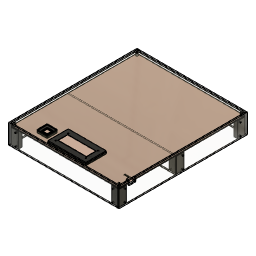
Case (Autodesk Fusion 360 design; units mm, degrees)
Autodesk Fusion 360 part; units mm, degrees
(part 1 of 2)
sketch "Sketch1" plane through (0, 0, 0) normal (0, 0, 1) x (1, 0, 0) in component "PCB"
  line L0 (-131, 153.5) -> (131, 153.5) construction
  line L1 (131, 153.5) -> (131, -153.5) construction
  line L2 (131, -153.5) -> (-131, -153.5) construction
  line L3 (-131, -153.5) -> (-131, 153.5) construction
  line L4 (-131, 153.5) -> (131, -153.5) construction
  line L5 (131, 153.5) -> (-131, -153.5) construction
  line L6 (-135, 157.5) -> (135, 157.5)
  line L7 (135, 157.5) -> (135, -157.5)
  line L8 (135, -157.5) -> (-135, -157.5)
  line L9 (-135, -157.5) -> (-135, 157.5)
  line L10 (-135, 157.5) -> (135, -157.5) construction
  line L11 (135, 157.5) -> (-135, -157.5) construction
  circle A0 centre (-131, 153.5) radius 1.6
  circle A1 centre (131, 153.5) radius 1.6
  circle A2 centre (-131, -153.5) radius 1.6
  circle A3 centre (131, -153.5) radius 1.6
  line L12 (135, -127.52) -> (128, -127.52) construction
  line L13 (128, -127.52) -> (128, -123.02)
  line L14 (128, -123.02) -> (135, -123.02)
  line L15 (128, -132.02) -> (135, -132.02)
  line L16 (128, -127.52) -> (128, -132.02)
  line L17 (122.64, -122.688) -> (112.36, -122.688)
  line L18 (112.36, -122.688) -> (112.36, -120.028)
  line L19 (112.36, -120.028) -> (122.64, -120.028)
  line L20 (122.64, -120.028) -> (122.64, -122.688)
  line L21 (122.64, -122.688) -> (112.36, -120.028) construction
  line L22 (112.36, -122.688) -> (122.64, -120.028) construction
  circle A4 centre (113.69, -121.358) radius 0.5
  circle A5 centre (116.23, -121.358) radius 0.5
  circle A6 centre (118.77, -121.358) radius 0.5
  circle A7 centre (121.31, -121.358) radius 0.5
  line L23 (113.69, -121.358) -> (116.23, -121.358) construction
  line L24 (116.23, -121.358) -> (118.77, -121.358) construction
  line L25 (118.77, -121.358) -> (121.31, -121.358) construction
  line L26 (121.31, -121.358) -> (122.64, -121.358) construction
  line L27 (113.69, -121.358) -> (112.36, -121.358) construction
  line L28 (-40, -109.858) -> (40, -109.858)
  line L29 (40, -109.858) -> (40, -145.858)
  line L30 (40, -145.858) -> (-40, -145.858)
  line L31 (-40, -145.858) -> (-40, -109.858)
  line L32 (-40, -109.858) -> (40, -145.858) construction
  line L33 (40, -109.858) -> (-40, -145.858) construction
  line L34 (-35.35, -115.958) -> (35.35, -115.958)
  line L35 (35.35, -115.958) -> (35.35, -139.758)
  line L36 (35.35, -139.758) -> (-35.35, -139.758)
  line L37 (-35.35, -139.758) -> (-35.35, -115.958)
  line L38 (-35.35, -115.958) -> (35.35, -139.758) construction
  line L39 (35.35, -115.958) -> (-35.35, -139.758) construction
  line L40 (-37.7, -112.158) -> (37.7, -112.158) construction
  line L41 (37.7, -112.158) -> (37.7, -143.558) construction
  line L42 (37.7, -143.558) -> (-37.7, -143.558) construction
  line L43 (-37.7, -143.558) -> (-37.7, -112.158) construction
  line L44 (-37.7, -112.158) -> (37.7, -143.558) construction
  line L45 (37.7, -112.158) -> (-37.7, -143.558) construction
  circle A8 centre (-37.7, -112.158) radius 1.4
  circle A9 centre (37.7, -112.158) radius 1.4
  circle A10 centre (37.7, -143.558) radius 1.4
  circle A11 centre (-37.7, -143.558) radius 1.4
  point P0 (117.5, -121.358)
  point P1 (0, -127.858)
  point P2 (0, -127.858)
  point P3 (0, -127.858)
  dimension "d1" = 262
  dimension "d2" = 307
  dimension "d3" = 270
  dimension "d4" = 315
  dimension "d5" = 3.2
  dimension "d8" = 29.98
  dimension "d9" = 9
  dimension "d10" = 7
  dimension "d17" = 10.28
  dimension "d18" = 2.66
  dimension "d19" = 2.54
  dimension "d20" = 1
  dimension "d21" = 36.142
  dimension "d22" = 17.5
  dimension "d30" = 29.642
  dimension "d31" = 135
  dimension "d32" = 80
  dimension "d33" = 36
  dimension "d34" = 70.7
  dimension "d35" = 23.8
  dimension "d279" = 75.4
  dimension "d280" = 31.4
  dimension "d281" = 2.8
  constraint horizontal L0
  constraint perpendicular L0 L1
  constraint parallel L0 L2
  constraint parallel L1 L3
  constraint coincident L4 origin
  constraint coincident L5 origin
  constraint horizontal L6
  constraint perpendicular L6 L7
  constraint parallel L6 L8
  constraint parallel L7 L9
  constraint coincident L10 origin
  constraint coincident L11 origin
  constraint coincident L0.start L3.end
  constraint coincident L0.end L1.start
  constraint coincident L2.end L3.start
  constraint coincident L1.end L2.start
  constraint equal A1 A3
  constraint equal A2 A3
  constraint equal A0 A2
  constraint coincident L7 L12.start
  constraint perpendicular L1 L12
  constraint perpendicular L12 L13
  constraint coincident L7 L14.end
  constraint perpendicular L7 L14
  constraint symmetric L13.start L12 L16.start
  constraint symmetric L12 L13.end L15.start
  constraint symmetric L12 L14.end L15.end
  constraint horizontal L17
  constraint perpendicular L17 L18
  constraint parallel L17 L19
  constraint parallel L18 L20
  constraint coincident L21 P0
  constraint coincident L22 P0
  constraint coincident A4.centre L23.start
  constraint horizontal L23
  constraint coincident A5.centre L23.end
  constraint equal A4 A5
  constraint equal A5 A6
  constraint equal A6 A7
  constraint parallel L23 L24
  constraint parallel L23 L25
  constraint parallel L25 L26
  constraint coincident A6.centre L24.end
  constraint coincident A7.centre L25.end
  constraint equal L23 L24
  constraint equal L24 L25
  constraint parallel L23 L27
  constraint equal L26 L27
  constraint midpoint L18 L27.end
  constraint midpoint L20 L26.end
  constraint horizontal L28
  constraint perpendicular L28 L29
  constraint parallel L28 L30
  constraint parallel L29 L31
  constraint coincident L32 P3
  constraint coincident L33 P3
  constraint horizontal L34
  constraint perpendicular L34 L35
  constraint parallel L34 L36
  constraint parallel L35 L37
  constraint coincident L38 P3
  constraint coincident L39 P3
  constraint coincident P3 P2
  constraint horizontal L40
  constraint perpendicular L40 L41
  constraint parallel L40 L42
  constraint parallel L41 L43
  constraint coincident L44 P3
  constraint coincident L45 P3
  constraint coincident L40.start L43.end
  constraint coincident L40.end L41.start
  constraint coincident L41.end L42.start
  constraint coincident L42.end L43.start
  constraint equal A8 A11
  constraint equal A8 A9
  constraint equal A9 A10
  measures "d1" distance of L1.end L2.end
  measures "d2" distance of L0.end L1.end
  measures "d3" distance of L7.end L8.end
  measures "d4" distance of L6.end L7.end
  measures "d5" diameter of A0
  measures "d8" distance of L7.end L12.start
  measures "d9" distance of L14 L15
  measures "d10" distance of L13.end L14.end
  measures "d17" distance of L18.end L19.end
  measures "d18" distance of L17.end L18.end
  measures "d19" distance of A4.centre A5.centre
  measures "d20" diameter of A7
  measures "d21" distance of L8 P0
  measures "d22" distance of L7 P0
  measures "d30" distance of L8 P3
  measures "d31" distance of L9 P3
  measures "d32" distance of L28.start L28.end
  measures "d33" distance of L28.end L29.end
  measures "d34" distance of L35.end L36.end
  measures "d35" distance of L34.end L35.end
  measures "d279" distance of L41.end L42.end
  measures "d280" distance of L40.end L41.end
  measures "d281" diameter of A8
extrude "Extrude1" add sketch "Sketch1" along normal blind 1.6 contours L6 L7 L8 L9 L13 L14 L15 L16 makes body 1 in component "PCB"
extrude "Extrude2" add sketch "Sketch1" along normal blind 5 contours L7 L13 L14 L15 L16 bodies 1 in component "PCB"
extrude "Extrude3" add sketch "Sketch1" along normal blind 4 contours L28 L29 L30 L31 bodies 1 in component "PCB"
extrude "Extrude4" add sketch "Sketch1" along normal blind 11 contours L34 L35 L36 L37 bodies 1 in component "PCB"
sketch "Sketch1 (2)" plane through (0, 0, 0) normal (0, 0, 1) x (1, 0, 0) in component "Corner"
  circle A0 centre (0, 0) radius 2.3
  line L0 (0, 0) -> (0, -9.2) construction
  line L1 (0, 0) -> (9.2, 0) construction
  circle A1 centre (0, -9.2) radius 2.3
  circle A2 centre (9.2, 0) radius 2.3
  line L2 (-4.6, 4.6) -> (-4.6, -13.8)
  line L3 (-4.6, -13.8) -> (4.6, -13.8)
  line L4 (4.6, -13.8) -> (4.6, -4.6)
  line L5 (4.6, -4.6) -> (13.8, -4.6)
  line L6 (13.8, -4.6) -> (13.8, 4.6)
  line L7 (13.8, 4.6) -> (-4.6, 4.6)
  line L8 (4.6, 0) -> (4.6, 4.6) construction
  line L9 (4.6, 0) -> (4.6, -4.6) construction
  line L10 (0, -4.6) -> (4.6, -4.6) construction
  line L11 (0, -4.6) -> (-4.6, -4.6) construction
  line L12 (9.2, 0) -> (13.8, 0) construction
  line L13 (0, -9.2) -> (0, -13.8) construction
  dimension "d41" = 4.6
  dimension "d42" = 9.2
  dimension "d43" = 4.6
  dimension "d44" = 4.6
  constraint coincident A0.centre L0.start
  constraint vertical L0
  constraint perpendicular L0 L1
  constraint equal L0 L1
  constraint coincident L0.end A1.centre
  constraint coincident L1.end A2.centre
  constraint equal A0 A2
  constraint equal A1 A2
  constraint vertical L2
  constraint perpendicular L2 L3
  constraint perpendicular L3 L4
  constraint perpendicular L4 L5
  constraint perpendicular L5 L6
  constraint perpendicular L6 L7
  constraint coincident L2.start L7.end
  constraint midpoint L1 L8.start
  constraint coincident L7 L8.end
  constraint perpendicular L7 L8
  constraint coincident L5 L4.end
  constraint perpendicular L5 L9
  constraint midpoint L0 L10.start
  constraint coincident L4 L5.start
  constraint perpendicular L4 L10
  constraint coincident L2 L11.end
  constraint perpendicular L2 L11
  constraint coincident L4.end L5.start
  constraint midpoint L6 L12.end
  constraint midpoint L3 L13.end
  constraint equal L11 L13
  constraint equal L12 L13
  measures "d41" diameter of A0
  measures "d42" distance of A0.centre L0.end
  measures "d43" distance of L8.start L8.end
  measures "d44" distance of L10.start L11.end
extrude "Extrude1'" add sketch "Sketch1 (2)" along normal blind 9 separate body contours A1 | A2 | L2 L3 L4 L5 L6 L7 makes body 2 in component "Corner"
extrude "Extrude2'" add sketch "Sketch1 (2)" along normal blind 3 contours A0 bodies 2 in component "Corner"
sketch "Sketch2" plane through (-4.6, 0, 0) normal (-1, 0, 0) x (0, -1, 0) in component "Corner"
  line L0 (-4.6, 0) -> (13.8, 0)
  line L1 (13.8, 0) -> (13.8, 9)
  line L2 (13.8, 9) -> (-4.6, 9)
  line L3 (-4.6, 9) -> (-4.6, 0)
  line L4 (11.5, 0) -> (6.9, 0)
  line L5 (13.8, 4.5) -> (9.2, 4.5) construction
  line L6 (9.2, 0) -> (9.2, 4.5) construction
  circle A0 centre (9.2, 4.5) radius 1.45
  dimension "d49" = 2.9
  constraint midpoint L1 L5.start
  constraint perpendicular L1 L5
  constraint midpoint L4 L6.start
  constraint perpendicular L4 L6
  constraint coincident L5.end L6.end
  measures "d49" diameter of A0
extrude "Extrude3'" cut sketch "Sketch2" against normal blind 6 contours A0 bodies 2 in component "Corner"
sketch "Sketch3" plane through (0, 4.6, 0) normal (0, 1, 0) x (-1, 0, 0) in component "Corner"
  line L0 (-13.8, 0) -> (4.6, 0)
  line L1 (4.6, 0) -> (4.6, 9)
  line L2 (4.6, 9) -> (-13.8, 9)
  line L3 (-13.8, 9) -> (-13.8, 0)
  line L4 (-6.9, 0) -> (-11.5, 0)
  line L5 (-13.8, 4.5) -> (-9.2, 4.5) construction
  line L6 (-9.2, 0) -> (-9.2, 4.5) construction
  circle A0 centre (-9.2, 4.5) radius 1.45
  dimension "d52" = 2.9
  constraint midpoint L3 L5.start
  constraint perpendicular L3 L5
  constraint midpoint L4 L6.start
  constraint perpendicular L4 L6
  constraint coincident L5.end L6.end
  measures "d52" diameter of A0
extrude "Extrude4'" cut sketch "Sketch3" against normal blind 6 contours A0 bodies 2 in component "Corner"
sketch "Sketch1 (3)" plane through (0, 0, 0) normal (0, 0, 1) x (1, 0, 0) in component "Washer"
  circle A0 centre (0, 0) radius 1.6
  circle A1 centre (0, 0) radius 2.6
  dimension "d55" = 3.2
  dimension "d56" = 1
  constraint coincident A0.centre A1.centre
  measures "d55" diameter of A0
extrude "Extrude1''" add sketch "Sketch1 (3)" along normal blind 1 separate body makes body 3 in component "Washer"
sketch "Sketch1 (4)" plane through (0, 0, 0) normal (0, 0, 1) x (1, 0, 0) in component "PlateWasher"
  circle A0 centre (0, 0) radius 1.6
  circle A1 centre (0, 0) radius 2.6
  dimension "d59" = 3.2
  dimension "d60" = 1
  constraint coincident A0.centre A1.centre
  measures "d59" diameter of A0
extrude "Extrude1'''" add sketch "Sketch1 (4)" along normal blind 4 separate body makes body 4 in component "PlateWasher"
move_face "OffsetFaces1" offset 30 1 faces at (4.6, 1.5333, 0) on bodies 2 in component "Corner"
sketch "Sketch5" plane through (0, 4.6, 0) normal (0, 1, 0) x (-1, 0, 0) in component "Corner"
  circle A0 centre (-9.2, 4.5) radius 1.45
  line L0 (-13.8, -30) -> (4.6, -30)
  line L1 (4.6, -30) -> (4.6, 9)
  line L2 (4.6, 9) -> (-13.8, 9)
  line L3 (-13.8, 9) -> (-13.8, -30)
  line L4 (-9.2, 4.5) -> (-9.2, 9) construction
  line L5 (-9.2, -30) -> (-9.2, -25.5) construction
  circle A1 centre (-9.2, -25.5) radius 1.45
  line L6 (-9.2, -25.5) -> (-9.2, 4.5) construction
  constraint coincident A0.centre L4.start
  constraint coincident L2 L4.end
  constraint perpendicular L2 L4
  constraint coincident L0 L5.start
  constraint perpendicular L0 L5
  constraint coincident L5.end A1.centre
  constraint equal A0 A1
  constraint equal L4 L5
  constraint vertical L6
extrude "Extrude6" cut sketch "Sketch5" against normal up to surface (6 mm away) contours A1 bodies 2 in component "Corner"
sketch "Sketch6" plane through (-4.6, 0, 0) normal (-1, 0, 0) x (0, -1, 0) in component "Corner"
  circle A0 centre (9.2, 4.5) radius 1.45
  line L0 (-4.6, -30) -> (13.8, -30)
  line L1 (13.8, -30) -> (13.8, 9)
  line L2 (13.8, 9) -> (-4.6, 9)
  line L3 (-4.6, 9) -> (-4.6, -30)
  line L4 (9.2, 4.5) -> (9.2, 9) construction
  line L5 (9.2, -30) -> (9.2, -25.5) construction
  line L6 (9.2, -25.5) -> (9.2, 4.5) construction
  circle A1 centre (9.2, -25.5) radius 1.45
  constraint coincident A0.centre L4.start
  constraint coincident L2 L4.end
  constraint perpendicular L2 L4
  constraint coincident L0 L5.start
  constraint perpendicular L0 L5
  constraint parallel L4 L6
  constraint equal L4 L5
  constraint coincident L5.end L6.start
  constraint equal A0 A1
extrude "Extrude7" cut sketch "Sketch6" against normal up to surface (6 mm away) contours A1 bodies 2 in component "Corner"
sketch "Sketch1 (5)" plane through (0, -158.1, 0) normal (0, -1, 0) x (1, 0, 0) in component "Panel1"
  circle A0 centre (-121.8, -35.5) radius 1.45
  circle A1 centre (-121.8, -5.5) radius 1.45
  line L0 (-135.6, -40) -> (-117.2, -40)
  line L1 (-117.2, -40) -> (-117.2, -1)
  line L2 (-117.2, -1) -> (-135.6, -1)
  line L3 (-135.6, -1) -> (-135.6, -40)
  circle A2 centre (121.8, -35.5) radius 1.45
  circle A3 centre (121.8, -5.5) radius 1.45
  line L4 (117.2, -40) -> (135.6, -40)
  line L5 (135.6, -40) -> (135.6, -1)
  line L6 (135.6, -1) -> (117.2, -1)
  line L7 (117.2, -1) -> (117.2, -40)
  line L8 (-117.2, -40) -> (117.2, -40)
  line L9 (-128.4, 5.6) -> (-133.6, 5.6)
  line L10 (-135.6, -1) -> (-135.6, 5.6)
  line L11 (-135.6, 5.6) -> (-133.6, 5.6) construction
  line L12 (-135.6, 5.6) -> (-135.6, 8.6)
  line L13 (135.6, -1) -> (135.6, 8.6)
  line L14 (135.6, 8.6) -> (-135.6, 8.6)
  circle A4 centre (-121.8, -5.5) radius 1.6
  circle A5 centre (-121.8, -35.5) radius 1.6
  circle A6 centre (121.8, -5.5) radius 1.6
  circle A7 centre (121.8, -35.5) radius 1.6
  dimension "d120" = 3
  dimension "d123" = 3.2
  constraint coincident L0.end L1.start
  constraint coincident L4.start L7.end
  constraint coincident L2.end L3.start
  constraint perpendicular L2 L10
  constraint coincident L9.end L11.end
  constraint perpendicular L10 L11
  constraint perpendicular L11 L12
  constraint coincident L5.end L6.start
  constraint perpendicular L6 L13
  constraint perpendicular L12 L14
  constraint concentric A1 A4
  constraint concentric A0 A5
  constraint concentric A3 A6
  constraint concentric A2 A7
  constraint equal A6 A7
  constraint equal A4 A6
  constraint equal A4 A5
  measures "d120" distance of L10.end L12.end
  measures "d123" diameter of A4
extrude "Extrude1''''" add sketch "Sketch1 (5)" along normal blind 3 separate body contours L0 L1 L2 L3 | L1 L2 L6 L7 L8 L10 L12 L13 L14 | L4 L5 L6 L7 makes body 5 in component "Panel1"
sketch "Sketch1 (6)" plane through (135.6, 0, 0) normal (1, 0, 0) x (0, 1, 0) in component "Panel2"
  circle A0 centre (-144.3, -35.5) radius 1.45
  circle A1 centre (-144.3, -5.5) radius 1.45
  line L0 (-158.1, -40) -> (-139.7, -40)
  line L1 (-139.7, -40) -> (-139.7, -1)
  line L2 (-139.7, -1) -> (-158.1, -1)
  line L3 (-158.1, -1) -> (-158.1, -40)
  circle A2 centre (144.3, -35.5) radius 1.45
  circle A3 centre (144.3, -5.5) radius 1.45
  line L4 (139.7, -40) -> (158.1, -40)
  line L5 (158.1, -40) -> (158.1, -1)
  line L6 (158.1, -1) -> (139.7, -1)
  line L7 (139.7, -1) -> (139.7, -40)
  line L8 (-158.1, -40) -> (-158.1, 8.6)
  line L9 (-158.1, 8.6) -> (-161.1, 8.6)
  line L10 (-161.1, 8.6) -> (-161.1, -40)
  line L11 (-161.1, -40) -> (-158.1, -40)
  line L12 (161.1, -40) -> (161.1, 8.6)
  line L13 (161.1, 8.6) -> (158.1, 8.6)
  line L14 (158.1, 8.6) -> (158.1, -40)
  line L15 (158.1, -40) -> (161.1, -40)
  line L16 (139.7, -40) -> (-139.7, -40)
  line L17 (-158.1, 8.6) -> (158.1, 8.6)
  line L18 (-157.5, 0) -> (157.5, 0)
  line L19 (157.5, 0) -> (157.5, 1.6)
  line L20 (157.5, 1.6) -> (-123.02, 1.6)
  line L21 (-123.02, 1.6) -> (-123.02, 5)
  line L22 (-123.02, 5) -> (-132.02, 5)
  line L23 (-132.02, 5) -> (-132.02, 1.6)
  line L24 (-132.02, 1.6) -> (-157.5, 1.6)
  line L25 (-157.5, 1.6) -> (-157.5, 0)
  line L26 (-132.02, 5) -> (-123.02, 5) construction
  line L27 (-123.02, 5) -> (-123.02, 1.6) construction
  line L28 (-123.02, 1.6) -> (-132.02, 1.6) construction
  line L29 (-132.02, 1.6) -> (-132.02, 5) construction
  line L30 (-136.02, 9) -> (-119.02, 9)
  line L31 (-119.02, 9) -> (-119.02, -2.4)
  line L32 (-119.02, -2.4) -> (-136.02, -2.4)
  line L33 (-136.02, -2.4) -> (-136.02, 9)
  circle A4 centre (-144.3, -5.5) radius 1.6
  circle A5 centre (-144.3, -35.5) radius 1.6
  circle A6 centre (144.3, -5.5) radius 1.6
  circle A7 centre (144.3, -35.5) radius 1.6
  line L34 (0, -40) -> (0, 8.6) construction
  circle A8 centre (0, -35.5) radius 1.6
  circle A9 centre (0, -5.5) radius 1.6
  line L35 (144.3, -5.5) -> (0, -5.5) construction
  line L36 (144.3, -35.5) -> (0, -35.5) construction
  dimension "d128" = -4
  dimension "d129" = 3.2
  constraint coincident L4.start L7.end
  constraint coincident L0.end L1.start
  constraint coincident L8.end L9.start
  constraint coincident L13.end L14.start
  constraint horizontal L26
  constraint vertical L27
  constraint horizontal L28
  constraint vertical L29
  constraint coincident L20.end L21.start
  constraint coincident L22.end L23.start
  constraint concentric A1 A4
  constraint concentric A0 A5
  constraint concentric A3 A6
  constraint concentric A2 A7
  constraint equal A6 A7
  constraint equal A4 A6
  constraint equal A4 A5
  constraint midpoint L16 L34.start
  constraint midpoint L17 L34.end
  constraint coincident L34 A8.centre
  constraint coincident L34 A9.centre
  constraint coincident A3.centre A6.centre
  constraint perpendicular L7 L35
  constraint coincident A2.centre A7.centre
  constraint parallel L4 L36
  constraint coincident A8.centre L36.end
  constraint coincident A9.centre L35.end
  constraint equal A8 A9
  constraint equal A7 A8
  measures "d129" diameter of A5
extrude "Extrude1'''''" add sketch "Sketch1 (6)" along normal blind 3 separate body contours L0 L1 L2 L3 L8 | L3 L8 L9 L10 L11 | L1 L2 L6 L7 L8 L14 L16 L17 L18 L19 L20 L24 L25 L31 L32 L33 | L4 L5 L6 L7 L14 | L5 L12 L13 L14 L15 | L18 L24 L25 L33 | L18 L19 L20 L31 makes body 6 in component "Panel2"
sketch "Sketch1 (7)" plane through (-135.6, 0, 0) normal (-1, 0, 0) x (0, -1, 0) in component "Panel3"
  circle A0 centre (-144.3, -35.5) radius 1.45
  circle A1 centre (-144.3, -5.5) radius 1.45
  line L0 (-158.1, -40) -> (-139.7, -40)
  line L1 (-139.7, -40) -> (-139.7, -1)
  line L2 (-139.7, -1) -> (-158.1, -1)
  line L3 (-158.1, -1) -> (-158.1, -40)
  circle A2 centre (-144.3, -35.5) radius 1.6
  circle A3 centre (-144.3, -5.5) radius 1.6
  circle A4 centre (144.3, -35.5) radius 1.6
  circle A5 centre (144.3, -5.5) radius 1.6
  line L4 (119.02, -2.4) -> (119.02, 8.6)
  line L5 (119.02, 8.6) -> (-161.1, 8.6)
  line L6 (-161.1, 8.6) -> (-161.1, -40)
  line L7 (-161.1, -40) -> (161.1, -40)
  line L8 (161.1, -40) -> (161.1, 8.6)
  line L9 (161.1, 8.6) -> (136.02, 8.6)
  line L10 (136.02, 8.6) -> (136.02, -2.4)
  line L11 (136.02, -2.4) -> (119.02, -2.4)
  line L12 (136.02, 8.6) -> (119.02, 8.6)
  circle A6 centre (0, -5.5) radius 1.6
  circle A7 centre (0, -35.5) radius 1.6
  constraint coincident L9.end L10.start
  constraint coincident L4.end L5.start
extrude "Extrude1''''''" add sketch "Sketch1 (7)" along normal blind 3 separate body contours L0 L1 L2 L3 L7 | L1 L2 L3 L4 L5 L6 L7 L8 L9 L10 L11 | L4 L10 L11 L12 makes body 7 in component "Panel3"
sketch "Sketch1 (8)" plane through (0, 0, 5.6) normal (0, 0, 1) x (-1, 0, 0) in component "TopPanel"
  circle A0 centre (131, -153.5) radius 1.6
  circle A1 centre (131, -153.5) radius 2.6
  circle A2 centre (131, -153.5) radius 1.6
  circle A3 centre (-131, -153.5) radius 1.6
  circle A4 centre (-131, 153.5) radius 1.6
  circle A5 centre (131, 153.5) radius 1.6
  line L0 (135.6, 161.1) -> (135.6, -161.1)
  line L1 (135.6, -161.1) -> (138.6, -161.1)
  line L2 (138.6, -161.1) -> (138.6, 161.1)
  line L3 (138.6, 161.1) -> (135.6, 161.1)
  line L4 (-135.6, 158.1) -> (135.6, 158.1)
  line L5 (135.6, 158.1) -> (135.6, 161.1)
  line L6 (135.6, 161.1) -> (-135.6, 161.1)
  line L7 (-135.6, 161.1) -> (-135.6, 158.1)
  line L8 (-135.6, 136.02) -> (-135.6, 161.1)
  line L9 (-135.6, 161.1) -> (-138.6, 161.1)
  line L10 (-138.6, 161.1) -> (-138.6, 136.02)
  line L11 (-138.6, 136.02) -> (-135.6, 136.02)
  line L12 (-135.6, 119.02) -> (-135.6, 136.02)
  line L13 (-135.6, 136.02) -> (-138.6, 136.02)
  line L14 (-138.6, 136.02) -> (-138.6, 119.02)
  line L15 (-138.6, 119.02) -> (-135.6, 119.02)
  line L16 (-135.6, -161.1) -> (-135.6, 119.02)
  line L17 (-135.6, 119.02) -> (-138.6, 119.02)
  line L18 (-138.6, 119.02) -> (-138.6, -161.1)
  line L19 (-138.6, -161.1) -> (-135.6, -161.1)
  line L20 (-135.6, -161.1) -> (135.6, -161.1)
  line L21 (135.6, -161.1) -> (135.6, -158.1)
  line L22 (135.6, -158.1) -> (-135.6, -158.1)
  line L23 (-135.6, -158.1) -> (-135.6, -161.1)
  line L24 (-112.36, 120.028) -> (-122.64, 120.028)
  line L25 (-122.64, 120.028) -> (-122.64, 122.688)
  line L26 (-122.64, 122.688) -> (-112.36, 122.688)
  line L27 (-112.36, 122.688) -> (-112.36, 120.028)
  circle A6 centre (131, -153.5) radius 1.6
  circle A7 centre (-131, 153.5) radius 1.6
  circle A8 centre (131, 153.5) radius 1.6
  circle A9 centre (-131, -153.5) radius 1.6
  line L28 (-40, 145.858) -> (40, 145.858)
  line L29 (40, 145.858) -> (40, 109.858)
  line L30 (40, 109.858) -> (-40, 109.858)
  line L31 (-40, 109.858) -> (-40, 145.858)
  line L32 (-128, 123.02) -> (-135, 123.02)
  line L33 (-135, 123.02) -> (-135, -157.5)
  line L34 (-135, -157.5) -> (135, -157.5)
  line L35 (135, -157.5) -> (135, 157.5)
  line L36 (135, 157.5) -> (-135, 157.5)
  line L37 (-135, 157.5) -> (-135, 132.02)
  line L38 (-135, 132.02) -> (-128, 132.02)
  line L39 (-128, 132.02) -> (-128, 123.02)
  line L40 (-135.6, 136.02) -> (-135, 136.02)
  line L41 (-135.6, 119.02) -> (-135, 119.02)
  line L42 (-135, 123.02) -> (-135, 132.02)
  line L43 (-48, 153.858) -> (48, 153.858)
  line L44 (48, 153.858) -> (48, 101.858)
  line L45 (48, 101.858) -> (-48, 101.858)
  line L46 (-48, 101.858) -> (-48, 153.858)
  line L47 (87.5, 115.358) -> (62.5, 115.358)
  line L48 (62.5, 115.358) -> (62.5, 140.358)
  line L49 (62.5, 140.358) -> (87.5, 140.358)
  line L50 (87.5, 140.358) -> (87.5, 115.358)
  line L51 (87.5, 115.358) -> (62.5, 140.358) construction
  line L52 (62.5, 115.358) -> (87.5, 140.358) construction
  point P0 (75, 127.858)
  dimension "d136" = -8
  dimension "d138" = 25
  dimension "d139" = 60
  dimension "d140" = 29.642
  dimension "d174" = 25
  constraint coincident L8.start L11.end
  constraint coincident L37 L40.end
  constraint perpendicular L37 L40
  constraint coincident L12.start L15.end
  constraint coincident L33 L41.end
  constraint perpendicular L33 L41
  constraint coincident L32.end L33.start
  constraint coincident L37.end L38.start
  constraint horizontal L47
  constraint perpendicular L47 L48
  constraint parallel L47 L49
  constraint parallel L48 L50
  constraint coincident L51 P0
  constraint coincident L52 P0
  measures "d138" distance of L47.end L48.end
  measures "d139" distance of L35 P0
  measures "d140" distance of L36 P0
  measures "d174" distance of L48.end L49.end
extrude "Extrude1'''''''" add sketch "Sketch1 (8)" along normal blind 3 separate body contours A1 | L0 L4 L8 L16 L22 L33 L34 L35 L36 L37 L40 L41 | L12 L33 L37 L40 L41 L42 | L32 L33 L34 L35 L36 L37 L38 L39 | L32 L38 L39 L42 | L24 L25 L26 L27 makes body 8 in component "TopPanel"
sketch "Sketch2 (2)" plane through (0, 0, 1.6) normal (0, 0, 1) x (-1, 0, 0) in component "PCB"
  line L0 (-112.36, 120.028) -> (-122.64, 120.028)
  line L1 (-122.64, 120.028) -> (-122.64, 122.688)
  line L2 (-122.64, 122.688) -> (-112.36, 122.688)
  line L3 (-112.36, 122.688) -> (-112.36, 120.028)
  circle A0 centre (131, -153.5) radius 1.6
  circle A1 centre (-131, 153.5) radius 1.6
  circle A2 centre (131, 153.5) radius 1.6
  circle A3 centre (-131, -153.5) radius 1.6
  line L4 (-40, 145.858) -> (40, 145.858)
  line L5 (40, 145.858) -> (40, 109.858)
  line L6 (40, 109.858) -> (-40, 109.858)
  line L7 (-40, 109.858) -> (-40, 145.858)
  line L8 (-128, 123.02) -> (-135, 123.02)
  line L9 (-135, 123.02) -> (-135, -157.5)
  line L10 (-135, -157.5) -> (135, -157.5)
  line L11 (135, -157.5) -> (135, 157.5)
  line L12 (135, 157.5) -> (-135, 157.5)
  line L13 (-135, 157.5) -> (-135, 132.02)
  line L14 (-135, 132.02) -> (-128, 132.02)
  line L15 (-128, 132.02) -> (-128, 123.02)
  line L16 (120, -112.5) -> (120, -142.5)
  line L17 (120, -142.5) -> (90, -142.5)
  line L18 (90, -142.5) -> (60, -142.5)
  line L19 (90, -112.5) -> (90, -142.5)
  line L20 (60, -142.5) -> (30, -142.5)
  line L21 (60, -112.5) -> (60, -142.5)
  line L22 (30, -142.5) -> (0, -142.5)
  line L23 (30, -112.5) -> (30, -142.5)
  line L24 (0, -142.5) -> (-30, -142.5)
  line L25 (0, -112.5) -> (0, -142.5)
  line L26 (-30, -142.5) -> (-60, -142.5)
  line L27 (-30, -112.5) -> (-30, -142.5)
  line L28 (-60, -142.5) -> (-90, -142.5)
  line L29 (-60, -112.5) -> (-60, -142.5)
  line L30 (-90, -142.5) -> (-120, -142.5)
  line L31 (-90, -112.5) -> (-90, -142.5)
  line L32 (-60, -112.5) -> (-90, -112.5)
  line L33 (-90, -112.5) -> (-120, -112.5)
  line L34 (-60, -82.5) -> (-60, -112.5)
  line L35 (-30, -82.5) -> (-30, -112.5)
  line L36 (120, -82.5) -> (120, -112.5)
  line L37 (90, -112.5) -> (60, -112.5)
  line L38 (60, -82.5) -> (60, -112.5)
  line L39 (30, -112.5) -> (0, -112.5)
  line L40 (120, -112.5) -> (90, -112.5)
  line L41 (30, -82.5) -> (30, -112.5)
  line L42 (-30, -112.5) -> (-60, -112.5)
  line L43 (-90, -82.5) -> (-90, -112.5)
  line L44 (90, -82.5) -> (90, -112.5)
  line L45 (0, -82.5) -> (0, -112.5)
  line L46 (60, -112.5) -> (30, -112.5)
  line L47 (0, -112.5) -> (-30, -112.5)
  line L48 (-60, -82.5) -> (-90, -82.5)
  line L49 (-90, -82.5) -> (-120, -82.5)
  line L50 (-60, -52.5) -> (-60, -82.5)
  line L51 (-30, -52.5) -> (-30, -82.5)
  line L52 (120, -52.5) -> (120, -82.5)
  line L53 (90, -82.5) -> (60, -82.5)
  line L54 (60, -52.5) -> (60, -82.5)
  line L55 (30, -82.5) -> (0, -82.5)
  line L56 (120, -82.5) -> (90, -82.5)
  line L57 (30, -52.5) -> (30, -82.5)
  line L58 (-30, -82.5) -> (-60, -82.5)
  line L59 (-90, -52.5) -> (-90, -82.5)
  line L60 (90, -52.5) -> (90, -82.5)
  line L61 (0, -52.5) -> (0, -82.5)
  line L62 (60, -82.5) -> (30, -82.5)
  line L63 (0, -82.5) -> (-30, -82.5)
  line L64 (-60, -52.5) -> (-90, -52.5)
  line L65 (-90, -52.5) -> (-120, -52.5)
  line L66 (-60, -22.5) -> (-60, -52.5)
  line L67 (-30, -22.5) -> (-30, -52.5)
  line L68 (120, -22.5) -> (120, -52.5)
  line L69 (90, -52.5) -> (60, -52.5)
  line L70 (60, -22.5) -> (60, -52.5)
  line L71 (30, -52.5) -> (0, -52.5)
  line L72 (120, -52.5) -> (90, -52.5)
  line L73 (30, -22.5) -> (30, -52.5)
  line L74 (-30, -52.5) -> (-60, -52.5)
  line L75 (-90, -22.5) -> (-90, -52.5)
  line L76 (90, -22.5) -> (90, -52.5)
  line L77 (0, -22.5) -> (0, -52.5)
  line L78 (60, -52.5) -> (30, -52.5)
  line L79 (0, -52.5) -> (-30, -52.5)
  line L80 (-60, -22.5) -> (-90, -22.5)
  line L81 (-90, -22.5) -> (-120, -22.5)
  line L82 (-60, 7.5) -> (-60, -22.5)
  line L83 (-30, 7.5) -> (-30, -22.5)
  line L84 (120, 7.5) -> (120, -22.5)
  line L85 (90, -22.5) -> (60, -22.5)
  line L86 (60, 7.5) -> (60, -22.5)
  line L87 (30, -22.5) -> (0, -22.5)
  line L88 (120, -22.5) -> (90, -22.5)
  line L89 (30, 7.5) -> (30, -22.5)
  line L90 (-30, -22.5) -> (-60, -22.5)
  line L91 (-90, 7.5) -> (-90, -22.5)
  line L92 (90, 7.5) -> (90, -22.5)
  line L93 (0, 7.5) -> (0, -22.5)
  line L94 (60, -22.5) -> (30, -22.5)
  line L95 (0, -22.5) -> (-30, -22.5)
  line L96 (-60, 7.5) -> (-90, 7.5)
  line L97 (-90, 7.5) -> (-120, 7.5)
  line L98 (-60, 37.5) -> (-60, 7.5)
  line L99 (-30, 37.5) -> (-30, 7.5)
  line L100 (120, 37.5) -> (120, 7.5)
  line L101 (90, 7.5) -> (60, 7.5)
  line L102 (60, 37.5) -> (60, 7.5)
  line L103 (30, 7.5) -> (0, 7.5)
  line L104 (120, 7.5) -> (90, 7.5)
  line L105 (30, 37.5) -> (30, 7.5)
  line L106 (-30, 7.5) -> (-60, 7.5)
  line L107 (-90, 37.5) -> (-90, 7.5)
  line L108 (90, 37.5) -> (90, 7.5)
  line L109 (0, 37.5) -> (0, 7.5)
  line L110 (60, 7.5) -> (30, 7.5)
  line L111 (0, 7.5) -> (-30, 7.5)
  line L112 (-60, 37.5) -> (-90, 37.5)
  line L113 (-90, 37.5) -> (-120, 37.5)
  line L114 (-60, 67.5) -> (-60, 37.5)
  line L115 (-30, 67.5) -> (-30, 37.5)
  line L116 (120, 67.5) -> (120, 37.5)
  line L117 (90, 37.5) -> (60, 37.5)
  line L118 (60, 67.5) -> (60, 37.5)
  line L119 (30, 37.5) -> (0, 37.5)
  line L120 (120, 37.5) -> (90, 37.5)
  line L121 (30, 67.5) -> (30, 37.5)
  line L122 (-30, 37.5) -> (-60, 37.5)
  line L123 (-90, 67.5) -> (-90, 37.5)
  line L124 (90, 67.5) -> (90, 37.5)
  line L125 (0, 67.5) -> (0, 37.5)
  line L126 (60, 37.5) -> (30, 37.5)
  line L127 (0, 37.5) -> (-30, 37.5)
  line L128 (-60, 67.5) -> (-90, 67.5)
  line L129 (-90, 67.5) -> (-120, 67.5)
  line L130 (-60, 97.5) -> (-60, 67.5)
  line L131 (-30, 97.5) -> (-30, 67.5)
  line L132 (120, 97.5) -> (120, 67.5)
  line L133 (90, 67.5) -> (60, 67.5)
  line L134 (60, 97.5) -> (60, 67.5)
  line L135 (30, 67.5) -> (0, 67.5)
  line L136 (120, 67.5) -> (90, 67.5)
  line L137 (30, 97.5) -> (30, 67.5)
  line L138 (-30, 67.5) -> (-60, 67.5)
  line L139 (-90, 97.5) -> (-90, 67.5)
  line L140 (90, 97.5) -> (90, 67.5)
  line L141 (0, 97.5) -> (0, 67.5)
  line L142 (60, 67.5) -> (30, 67.5)
  line L143 (0, 67.5) -> (-30, 67.5)
  line L144 (-120, -142.5) -> (-120, 67.5)
  line L145 (120, 97.5) -> (-90, 97.5)
  line L146 (-120, 97.5) -> (-120, 67.5)
  line L147 (-120, 97.5) -> (-90, 97.5)
  line L148 (-120, -142.5) -> (-135, -142.5) construction
  line L149 (120, -142.5) -> (135, -142.5) construction
  line L150 (0, -142.5) -> (0, -157.5) construction
  dimension "d141" = 30
  dimension "d144" = -30
  dimension "d145" = 0
  dimension "d148" = 0
  dimension "d149" = 30
  constraint perpendicular L10 L16
  constraint perpendicular L16 L17
  constraint equal L16 L17
  constraint perpendicular L139 L147
  constraint perpendicular L146 L147
  constraint coincident L9 L148.end
  constraint perpendicular L9 L148
  constraint coincident L11 L149.end
  constraint perpendicular L11 L149
  constraint coincident L10 L150.end
  constraint perpendicular L10 L150
  constraint equal L149 L150
  constraint equal L148 L150
  measures "d141" distance of L16.end L17.end
sketch "Sketch3 (2)" plane through (0, 0, 8.6) normal (0, 0, 1) x (-1, 0, 0) in component "TopPanel"
  circle A0 centre (131, 153.5) radius 1.6
  line L0 (62.5, 140.358) -> (87.5, 140.358)
  line L1 (87.5, 140.358) -> (87.5, 115.358)
  line L2 (87.5, 115.358) -> (62.5, 115.358)
  line L3 (62.5, 115.358) -> (62.5, 140.358)
  circle A1 centre (-131, 153.5) radius 1.6
  circle A2 centre (-131, -153.5) radius 1.6
  line L4 (48, 101.858) -> (-48, 101.858)
  line L5 (-48, 101.858) -> (-48, 153.858)
  line L6 (-48, 153.858) -> (48, 153.858)
  line L7 (48, 153.858) -> (48, 101.858)
  line L8 (-135.6, 158.1) -> (-135.6, -158.1)
  line L9 (-135.6, -158.1) -> (135.6, -158.1)
  line L10 (135.6, -158.1) -> (135.6, 158.1)
  line L11 (135.6, 158.1) -> (-135.6, 158.1)
  line L12 (30, -112.5) -> (30, -142.5)
  line L13 (0, -112.5) -> (0, -142.5)
  line L14 (90, -52.5) -> (60, -52.5)
  line L15 (-30, -112.5) -> (-60, -112.5)
  line L16 (120, -142.5) -> (90, -142.5)
  line L17 (-30, -82.5) -> (-30, -112.5)
  line L18 (60, -52.5) -> (60, -82.5)
  line L19 (-30, -112.5) -> (-30, -142.5)
  line L20 (60, -112.5) -> (30, -112.5)
  line L21 (-60, 37.5) -> (-60, 7.5)
  line L22 (-90, 67.5) -> (-90, 37.5)
  line L23 (-30, 97.5) -> (-30, 67.5)
  line L24 (-60, 67.5) -> (-90, 67.5)
  line L25 (-90, 37.5) -> (-120, 37.5)
  line L26 (-120, 97.5) -> (-90, 97.5)
  line L27 (-60, 97.5) -> (-60, 67.5)
  line L28 (-90, 7.5) -> (-120, 7.5)
  line L29 (-30, 67.5) -> (-30, 37.5)
  line L30 (60, 7.5) -> (30, 7.5)
  line L31 (-30, 7.5) -> (-30, -22.5)
  line L32 (0, 67.5) -> (-30, 67.5)
  line L33 (120, -82.5) -> (120, -112.5)
  line L34 (-60, -22.5) -> (-90, -22.5)
  line L35 (-60, -82.5) -> (-90, -82.5)
  line L36 (30, 7.5) -> (0, 7.5)
  line L37 (60, 7.5) -> (60, -22.5)
  line L38 (60, -22.5) -> (60, -52.5)
  line L39 (120, 7.5) -> (120, -22.5)
  line L40 (-90, 7.5) -> (-90, -22.5)
  line L41 (30, -82.5) -> (0, -82.5)
  line L42 (30, 7.5) -> (30, -22.5)
  line L43 (60, 37.5) -> (60, 7.5)
  line L44 (120, 7.5) -> (90, 7.5)
  line L45 (0, 7.5) -> (0, -22.5)
  line L46 (0, 7.5) -> (-30, 7.5)
  line L47 (120, 67.5) -> (120, 37.5)
  line L48 (120, 97.5) -> (-90, 97.5)
  line L49 (30, -112.5) -> (0, -112.5)
  line L50 (30, 97.5) -> (30, 67.5)
  line L51 (30, -22.5) -> (0, -22.5)
  line L52 (30, -52.5) -> (0, -52.5)
  line L53 (0, 37.5) -> (-30, 37.5)
  line L54 (30, -142.5) -> (0, -142.5)
  line L55 (-60, -142.5) -> (-90, -142.5)
  line L56 (60, -82.5) -> (60, -112.5)
  line L57 (90, 7.5) -> (90, -22.5)
  line L58 (0, 37.5) -> (0, 7.5)
  line L59 (30, -82.5) -> (30, -112.5)
  line L60 (0, 97.5) -> (0, 67.5)
  line L61 (90, 67.5) -> (60, 67.5)
  line L62 (-30, 37.5) -> (-30, 7.5)
  line L63 (-60, 7.5) -> (-90, 7.5)
  line L64 (-90, 97.5) -> (-90, 67.5)
  line L65 (120, 67.5) -> (90, 67.5)
  line L66 (120, 37.5) -> (90, 37.5)
  line L67 (90, 37.5) -> (60, 37.5)
  line L68 (-60, 7.5) -> (-60, -22.5)
  line L69 (60, 37.5) -> (30, 37.5)
  line L70 (120, 37.5) -> (120, 7.5)
  line L71 (120, 97.5) -> (120, 67.5)
  line L72 (60, 97.5) -> (60, 67.5)
  line L73 (90, 97.5) -> (90, 67.5)
  line L74 (90, 67.5) -> (90, 37.5)
  line L75 (0, 67.5) -> (0, 37.5)
  line L76 (30, 37.5) -> (0, 37.5)
  line L77 (-120, -142.5) -> (-120, 67.5)
  line L78 (30, 37.5) -> (30, 7.5)
  line L79 (-90, 67.5) -> (-120, 67.5)
  line L80 (-60, 67.5) -> (-60, 37.5)
  line L81 (-60, 37.5) -> (-90, 37.5)
  line L82 (-30, 7.5) -> (-60, 7.5)
  line L83 (-90, 37.5) -> (-90, 7.5)
  line L84 (-30, 67.5) -> (-60, 67.5)
  line L85 (-120, 97.5) -> (-120, 67.5)
  line L86 (90, 7.5) -> (60, 7.5)
  line L87 (60, 67.5) -> (30, 67.5)
  line L88 (90, 37.5) -> (90, 7.5)
  line L89 (30, 67.5) -> (0, 67.5)
  line L90 (30, 67.5) -> (30, 37.5)
  line L91 (60, 67.5) -> (60, 37.5)
  line L92 (-30, 37.5) -> (-60, 37.5)
  line L93 (30, -22.5) -> (30, -52.5)
  line L94 (-30, -22.5) -> (-60, -22.5)
  line L95 (-90, -82.5) -> (-90, -112.5)
  line L96 (-30, -82.5) -> (-60, -82.5)
  line L97 (0, -112.5) -> (-30, -112.5)
  line L98 (90, -142.5) -> (60, -142.5)
  line L99 (90, -52.5) -> (90, -82.5)
  line L100 (90, -112.5) -> (60, -112.5)
  line L101 (-90, -112.5) -> (-120, -112.5)
  line L102 (-60, -52.5) -> (-90, -52.5)
  line L103 (-90, -82.5) -> (-120, -82.5)
  line L104 (0, -52.5) -> (0, -82.5)
  line L105 (0, -82.5) -> (0, -112.5)
  line L106 (-60, -52.5) -> (-60, -82.5)
  line L107 (-30, -52.5) -> (-60, -52.5)
  line L108 (0, -22.5) -> (-30, -22.5)
  line L109 (60, -82.5) -> (30, -82.5)
  line L110 (90, -82.5) -> (60, -82.5)
  line L111 (-60, -82.5) -> (-60, -112.5)
  line L112 (120, -52.5) -> (120, -82.5)
  line L113 (120, -112.5) -> (120, -142.5)
  line L114 (120, -52.5) -> (90, -52.5)
  line L115 (120, -82.5) -> (90, -82.5)
  line L116 (0, -22.5) -> (0, -52.5)
  line L117 (0, -52.5) -> (-30, -52.5)
  line L118 (90, -112.5) -> (90, -142.5)
  line L119 (-30, -22.5) -> (-30, -52.5)
  line L120 (120, -22.5) -> (120, -52.5)
  line L121 (-90, -52.5) -> (-90, -82.5)
  line L122 (60, -52.5) -> (30, -52.5)
  line L123 (-90, -112.5) -> (-90, -142.5)
  line L124 (0, -142.5) -> (-30, -142.5)
  line L125 (120, -112.5) -> (90, -112.5)
  line L126 (-90, -22.5) -> (-90, -52.5)
  line L127 (0, -82.5) -> (-30, -82.5)
  line L128 (60, -112.5) -> (60, -142.5)
  line L129 (60, -22.5) -> (30, -22.5)
  line L130 (90, -82.5) -> (90, -112.5)
  line L131 (-90, -22.5) -> (-120, -22.5)
  line L132 (-90, -52.5) -> (-120, -52.5)
  line L133 (90, -22.5) -> (90, -52.5)
  line L134 (120, -22.5) -> (90, -22.5)
  line L135 (-30, -52.5) -> (-30, -82.5)
  line L136 (-60, -22.5) -> (-60, -52.5)
  line L137 (90, -22.5) -> (60, -22.5)
  line L138 (-60, -112.5) -> (-90, -112.5)
  line L139 (-60, -112.5) -> (-60, -142.5)
  line L140 (-90, -142.5) -> (-120, -142.5)
  line L141 (60, -142.5) -> (30, -142.5)
  line L142 (30, -52.5) -> (30, -82.5)
  line L143 (-30, -142.5) -> (-60, -142.5)
  line L144 (120, -142.5) -> (135.6, -142.5) construction
  line L145 (-120, -142.5) -> (-135.6, -142.5) construction
  line L146 (0, -142.5) -> (0, -158.1) construction
  line L147 (120, 88.9286) -> (111.4286, 97.5)
  line L148 (120, 80.3571) -> (102.8571, 97.5)
  line L149 (120, 71.7857) -> (94.2857, 97.5)
  line L150 (115.7143, 67.5) -> (90, 93.2143)
  line L151 (98.5714, 67.5) -> (90, 76.0714)
  line L152 (107.1429, 67.5) -> (90, 84.6429)
  line L153 (115.7143, 93.2143) -> (111.4286, 88.9286) construction
  line L154 (111.4286, 88.9286) -> (107.1429, 84.6429) construction
  line L155 (107.1429, 84.6429) -> (102.8571, 80.3571) construction
  line L156 (102.8571, 80.3571) -> (98.5714, 76.0714) construction
  line L157 (98.5714, 76.0714) -> (94.2857, 71.7857) construction
  line L158 (94.2857, 71.7857) -> (90, 67.5) construction
  line L159 (115.7143, 93.2143) -> (120, 97.5) construction
  line L160 (60, 88.9286) -> (51.4286, 97.5)
  line L161 (60, 80.3571) -> (42.8571, 97.5)
  line L162 (60, 71.7857) -> (34.2857, 97.5)
  line L163 (55.7143, 67.5) -> (30, 93.2143)
  line L164 (47.1429, 67.5) -> (30, 84.6429)
  line L165 (38.5714, 67.5) -> (30, 76.0714)
  line L166 (0, 88.9286) -> (-8.5714, 97.5)
  line L167 (0, 80.3571) -> (-17.1429, 97.5)
  line L168 (0, 71.7857) -> (-25.7143, 97.5)
  line L169 (-4.2857, 67.5) -> (-30, 93.2143)
  line L170 (-12.8571, 67.5) -> (-30, 84.6429)
  line L171 (-21.4286, 67.5) -> (-30, 76.0714)
  line L172 (-60, 88.9286) -> (-68.5714, 97.5)
  line L173 (-60, 80.3571) -> (-77.1429, 97.5)
  line L174 (-60, 71.7857) -> (-85.7143, 97.5)
  line L175 (-64.2857, 67.5) -> (-90, 93.2143)
  line L176 (-72.8571, 67.5) -> (-90, 84.6429)
  line L177 (-81.4286, 67.5) -> (-90, 76.0714)
  line L178 (120, 28.9286) -> (111.4286, 37.5)
  line L179 (120, 20.3571) -> (102.8571, 37.5)
  line L180 (120, 11.7857) -> (94.2857, 37.5)
  line L181 (115.7143, 7.5) -> (90, 33.2143)
  line L182 (107.1429, 7.5) -> (90, 24.6429)
  line L183 (98.5714, 7.5) -> (90, 16.0714)
  line L184 (60, 28.9286) -> (51.4286, 37.5)
  line L185 (60, 20.3571) -> (42.8571, 37.5)
  line L186 (60, 11.7857) -> (34.2857, 37.5)
  line L187 (55.7143, 7.5) -> (30, 33.2143)
  line L188 (47.1429, 7.5) -> (30, 24.6429)
  line L189 (38.5714, 7.5) -> (30, 16.0714)
  line L190 (0, 28.9286) -> (-8.5714, 37.5)
  line L191 (0, 20.3571) -> (-17.1429, 37.5)
  line L192 (0, 11.7857) -> (-25.7143, 37.5)
  line L193 (-4.2857, 7.5) -> (-30, 33.2143)
  line L194 (-12.8571, 7.5) -> (-30, 24.6429)
  line L195 (-21.4286, 7.5) -> (-30, 16.0714)
  line L196 (-60, 28.9286) -> (-68.5714, 37.5)
  line L197 (-60, 20.3571) -> (-77.1429, 37.5)
  line L198 (-60, 11.7857) -> (-85.7143, 37.5)
  line L199 (-64.2857, 7.5) -> (-90, 33.2143)
  line L200 (-72.8571, 7.5) -> (-90, 24.6429)
  line L201 (-81.4286, 7.5) -> (-90, 16.0714)
  line L202 (120, -31.0714) -> (111.4286, -22.5)
  line L203 (120, -39.6429) -> (102.8571, -22.5)
  line L204 (120, -48.2143) -> (94.2857, -22.5)
  line L205 (115.7143, -52.5) -> (90, -26.7857)
  line L206 (107.1429, -52.5) -> (90, -35.3571)
  line L207 (98.5714, -52.5) -> (90, -43.9286)
  line L208 (60, -31.0714) -> (51.4286, -22.5)
  line L209 (60, -39.6429) -> (42.8571, -22.5)
  line L210 (60, -48.2143) -> (34.2857, -22.5)
  line L211 (55.7143, -52.5) -> (30, -26.7857)
  line L212 (47.1429, -52.5) -> (30, -35.3571)
  line L213 (38.5714, -52.5) -> (30, -43.9286)
  line L214 (0, -31.0714) -> (-8.5714, -22.5)
  line L215 (0, -39.6429) -> (-17.1429, -22.5)
  line L216 (0, -48.2143) -> (-25.7143, -22.5)
  line L217 (-4.2857, -52.5) -> (-30, -26.7857)
  line L218 (-12.8571, -52.5) -> (-30, -35.3571)
  line L219 (-21.4286, -52.5) -> (-30, -43.9286)
  line L220 (-60, -31.0714) -> (-68.5714, -22.5)
  line L221 (-60, -39.6429) -> (-77.1429, -22.5)
  line L222 (-60, -48.2143) -> (-85.7143, -22.5)
  line L223 (-64.2857, -52.5) -> (-90, -26.7857)
  line L224 (-72.8571, -52.5) -> (-90, -35.3571)
  line L225 (-81.4286, -52.5) -> (-90, -43.9286)
  line L226 (120, -91.0714) -> (111.4286, -82.5)
  line L227 (120, -99.6429) -> (102.8571, -82.5)
  line L228 (120, -108.2143) -> (94.2857, -82.5)
  line L229 (115.7143, -112.5) -> (90, -86.7857)
  line L230 (107.1429, -112.5) -> (90, -95.3571)
  line L231 (98.5714, -112.5) -> (90, -103.9286)
  line L232 (60, -91.0714) -> (51.4286, -82.5)
  line L233 (60, -99.6429) -> (42.8571, -82.5)
  line L234 (60, -108.2143) -> (34.2857, -82.5)
  line L235 (55.7143, -112.5) -> (30, -86.7857)
  line L236 (47.1429, -112.5) -> (30, -95.3571)
  line L237 (38.5714, -112.5) -> (30, -103.9286)
  line L238 (0, -91.0714) -> (-8.5714, -82.5)
  line L239 (0, -99.6429) -> (-17.1429, -82.5)
  line L240 (0, -108.2143) -> (-25.7143, -82.5)
  line L241 (-4.2857, -112.5) -> (-30, -86.7857)
  line L242 (-12.8571, -112.5) -> (-30, -95.3571)
  line L243 (-21.4286, -112.5) -> (-30, -103.9286)
  line L244 (-60, -91.0714) -> (-68.5714, -82.5)
  line L245 (-60, -99.6429) -> (-77.1429, -82.5)
  line L246 (-60, -108.2143) -> (-85.7143, -82.5)
  line L247 (-64.2857, -112.5) -> (-90, -86.7857)
  line L248 (-72.8571, -112.5) -> (-90, -95.3571)
  line L249 (-81.4286, -112.5) -> (-90, -103.9286)
  line L250 (81.4286, 67.5) -> (90, 58.9286)
  line L251 (90, 50.3571) -> (72.8571, 67.5)
  line L252 (90, 41.7857) -> (64.2857, 67.5)
  line L253 (60, 46.0714) -> (68.5714, 37.5)
  line L254 (77.1429, 37.5) -> (60, 54.6429)
  line L255 (85.7143, 37.5) -> (60, 63.2143)
  line L256 (85.7143, 63.2143) -> (81.4286, 58.9286) construction
  line L257 (81.4286, 58.9286) -> (77.1429, 54.6429) construction
  line L258 (77.1429, 54.6429) -> (72.8571, 50.3571) construction
  line L259 (72.8571, 50.3571) -> (68.5714, 46.0714) construction
  line L260 (68.5714, 46.0714) -> (64.2857, 41.7857) construction
  line L261 (64.2857, 41.7857) -> (60, 37.5) construction
  line L262 (85.7143, 63.2143) -> (90, 67.5) construction
  line L263 (21.4286, 67.5) -> (30, 58.9286)
  line L264 (30, 50.3571) -> (12.8571, 67.5)
  line L265 (30, 41.7857) -> (4.2857, 67.5)
  line L266 (25.7143, 37.5) -> (0, 63.2143)
  line L267 (17.1429, 37.5) -> (0, 54.6429)
  line L268 (0, 46.0714) -> (8.5714, 37.5)
  line L269 (-38.5714, 67.5) -> (-30, 58.9286)
  line L270 (-30, 50.3571) -> (-47.1429, 67.5)
  line L271 (-30, 41.7857) -> (-55.7143, 67.5)
  line L272 (-34.2857, 37.5) -> (-60, 63.2143)
  line L273 (-42.8571, 37.5) -> (-60, 54.6429)
  line L274 (-60, 46.0714) -> (-51.4286, 37.5)
  line L275 (-98.5714, 67.5) -> (-90, 58.9286)
  line L276 (-90, 50.3571) -> (-107.1429, 67.5)
  line L277 (-90, 41.7857) -> (-115.7143, 67.5)
  line L278 (-94.2857, 37.5) -> (-120, 63.2143)
  line L279 (-102.8571, 37.5) -> (-120, 54.6429)
  line L280 (-120, 46.0714) -> (-111.4286, 37.5)
  line L281 (81.4286, 7.5) -> (90, -1.0714)
  line L282 (90, -9.6429) -> (72.8571, 7.5)
  line L283 (90, -18.2143) -> (64.2857, 7.5)
  line L284 (85.7143, -22.5) -> (60, 3.2143)
  line L285 (77.1429, -22.5) -> (60, -5.3571)
  line L286 (60, -13.9286) -> (68.5714, -22.5)
  line L287 (21.4286, 7.5) -> (30, -1.0714)
  line L288 (30, -9.6429) -> (12.8571, 7.5)
  line L289 (30, -18.2143) -> (4.2857, 7.5)
  line L290 (25.7143, -22.5) -> (0, 3.2143)
  line L291 (17.1429, -22.5) -> (0, -5.3571)
  line L292 (0, -13.9286) -> (8.5714, -22.5)
  line L293 (-38.5714, 7.5) -> (-30, -1.0714)
  line L294 (-30, -9.6429) -> (-47.1429, 7.5)
  line L295 (-30, -18.2143) -> (-55.7143, 7.5)
  line L296 (-34.2857, -22.5) -> (-60, 3.2143)
  line L297 (-42.8571, -22.5) -> (-60, -5.3571)
  line L298 (-60, -13.9286) -> (-51.4286, -22.5)
  line L299 (-98.5714, 7.5) -> (-90, -1.0714)
  line L300 (-90, -9.6429) -> (-107.1429, 7.5)
  line L301 (-90, -18.2143) -> (-115.7143, 7.5)
  line L302 (-94.2857, -22.5) -> (-120, 3.2143)
  line L303 (-102.8571, -22.5) -> (-120, -5.3571)
  line L304 (-120, -13.9286) -> (-111.4286, -22.5)
  line L305 (81.4286, -52.5) -> (90, -61.0714)
  line L306 (90, -69.6429) -> (72.8571, -52.5)
  line L307 (90, -78.2143) -> (64.2857, -52.5)
  line L308 (85.7143, -82.5) -> (60, -56.7857)
  line L309 (77.1429, -82.5) -> (60, -65.3571)
  line L310 (60, -73.9286) -> (68.5714, -82.5)
  line L311 (21.4286, -52.5) -> (30, -61.0714)
  line L312 (30, -69.6429) -> (12.8571, -52.5)
  line L313 (30, -78.2143) -> (4.2857, -52.5)
  line L314 (25.7143, -82.5) -> (0, -56.7857)
  line L315 (17.1429, -82.5) -> (0, -65.3571)
  line L316 (0, -73.9286) -> (8.5714, -82.5)
  line L317 (-38.5714, -52.5) -> (-30, -61.0714)
  line L318 (-30, -69.6429) -> (-47.1429, -52.5)
  line L319 (-30, -78.2143) -> (-55.7143, -52.5)
  line L320 (-34.2857, -82.5) -> (-60, -56.7857)
  line L321 (-42.8571, -82.5) -> (-60, -65.3571)
  line L322 (-60, -73.9286) -> (-51.4286, -82.5)
  line L323 (-98.5714, -52.5) -> (-90, -61.0714)
  line L324 (-90, -69.6429) -> (-107.1429, -52.5)
  line L325 (-90, -78.2143) -> (-115.7143, -52.5)
  line L326 (-94.2857, -82.5) -> (-120, -56.7857)
  line L327 (-102.8571, -82.5) -> (-120, -65.3571)
  line L328 (-120, -73.9286) -> (-111.4286, -82.5)
  line L329 (81.4286, -112.5) -> (90, -121.0714)
  line L330 (90, -129.6429) -> (72.8571, -112.5)
  line L331 (90, -138.2143) -> (64.2857, -112.5)
  line L332 (85.7143, -142.5) -> (60, -116.7857)
  line L333 (77.1429, -142.5) -> (60, -125.3571)
  line L334 (60, -133.9286) -> (68.5714, -142.5)
  line L335 (21.4286, -112.5) -> (30, -121.0714)
  line L336 (30, -129.6429) -> (12.8571, -112.5)
  line L337 (30, -138.2143) -> (4.2857, -112.5)
  line L338 (25.7143, -142.5) -> (0, -116.7857)
  line L339 (17.1429, -142.5) -> (0, -125.3571)
  line L340 (0, -133.9286) -> (8.5714, -142.5)
  line L341 (-38.5714, -112.5) -> (-30, -121.0714)
  line L342 (-30, -129.6429) -> (-47.1429, -112.5)
  line L343 (-30, -138.2143) -> (-55.7143, -112.5)
  line L344 (-34.2857, -142.5) -> (-60, -116.7857)
  line L345 (-42.8571, -142.5) -> (-60, -125.3571)
  line L346 (-60, -133.9286) -> (-51.4286, -142.5)
  line L347 (-98.5714, -112.5) -> (-90, -121.0714)
  line L348 (-90, -129.6429) -> (-107.1429, -112.5)
  line L349 (-90, -138.2143) -> (-115.7143, -112.5)
  line L350 (-94.2857, -142.5) -> (-120, -116.7857)
  line L351 (-102.8571, -142.5) -> (-120, -125.3571)
  line L352 (-120, -133.9286) -> (-111.4286, -142.5)
  circle A3 centre (131, -153.5) radius 1.6
  point P0 (350, 0)
  dimension "d152" = -30
  dimension "d153" = 0
  dimension "d156" = 0
  dimension "d157" = 30
  dimension "d158" = 30
  dimension "d159" = 45
  dimension "d162" = -60
  dimension "d163" = -60
  dimension "d164" = 45
  dimension "d167" = -60
  dimension "d168" = -60
  constraint perpendicular L16 L113
  constraint equal L16 L113
  constraint perpendicular L26 L64
  constraint perpendicular L26 L85
  constraint vertical L113
  constraint coincident L10 L144.end
  constraint perpendicular L10 L144
  constraint coincident L8 L145.end
  constraint perpendicular L8 L145
  constraint coincident L9 L146.end
  constraint perpendicular L9 L146
  constraint equal L144 L145
  constraint equal L145 L146
  constraint coincident L71 L147.start
  constraint coincident L48 L147.end
  constraint coincident L71 L148.start
  constraint coincident L48 L148.end
  constraint parallel L147 L148
  constraint coincident L71 L149.start
  constraint coincident L48 L149.end
  constraint parallel L148 L149
  constraint coincident L65 L150.start
  constraint coincident L73 L150.end
  constraint parallel L149 L150
  constraint coincident L65 L151.start
  constraint coincident L73 L151.end
  constraint coincident L65 L152.start
  constraint coincident L73 L152.end
  constraint parallel L151 L152
  constraint parallel L150 L152
  constraint midpoint L147 L153.start
  constraint midpoint L148 L153.end
  constraint midpoint L149 L154.end
  constraint midpoint L150 L155.end
  constraint midpoint L152 L156.end
  constraint midpoint L151 L157.end
  constraint equal L153 L154
  constraint equal L154 L155
  constraint equal L155 L156
  constraint equal L156 L157
  constraint equal L158 L159
  constraint equal L157 L158
  constraint coincident L61 L250.start
  constraint coincident L74 L250.end
  constraint coincident L74 L251.start
  constraint coincident L61 L251.end